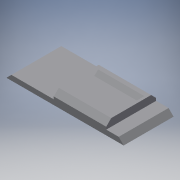
# Autodesk Inventor part: deksel token Nieuw bevestiging uitwendig
Saved by Autodesk Inventor 2018.3 (Build 223284000, 284)
## iProperties
Created: 2020-11-30
Part Number: deksel token Nieuw bevestiging uitwendig
Material: Generic
Document SubType Name: Modeling
Designer: Olivi
Density: 1 g/cm^3
Appearance: Default
Author: Olivi
## iProperties of the stored document deksel token Nieuw bevestiging uitwendig_3DPrint.ipt
Created: 2021-01-08
Part Number: deksel token Nieuw bevestiging uitwendig_3DPrint
Material: Generic
Document SubType Name: Modeling
Designer: daanv
Density: 1 g/cm^3
Appearance: Default
Author: daanv
Autodesk Inventor part; units mm, degrees
ref_plane "YZ Plane" through (0, 0, 0) normal (1, 0, 0) x (0, 1, 0)
ref_plane "XZ Plane" through (0, 0, 0) normal (0, 1, 0) x (-1, 0, 0)
ref_plane "XY Plane" through (0, 0, 0) normal (0, 0, 1) x (1, 0, 0)
sketch "Sketch1" plane through (0, 0, 0) normal (0, 0, 1) x (1, 0, 0)
  line L0 (0, 0) -> (43, 0)
  line L1 (43, 0) -> (43, 20)
  line L2 (43, 20) -> (0, 20)
  line L3 (0, 20) -> (0, 0)
  dimension "d0" = 43
  dimension "d1" = 20
  constraints: 8 end point, 2 parallel, 1 horizontal, 1 perpendicular
  measures "d0" distance of L2.end L1.end
  measures "d1" distance of L1.end L0.end
extrude "Extrusion1" add sketch "Sketch1" along normal blind 2
sketch "Sketch2" plane through (0, 0, 0) normal (0, -1, 0) x (1, 0, 0)
  line L0 (43, 0) -> (43, 2) projected
  line L1 (0, 0) -> (0, 2) projected
  line L2 (0, 0) -> (-2, 0)
  line L3 (-2, 0) -> (0, 2)
  line L4 (43, 0) -> (45, 0)
  line L5 (45, 0) -> (43, 2)
  dimension "d4" = 2
  dimension "d5" = 2
  constraints: 8 end point, 2 horizontal
  measures "d4" distance of L1.start L2.end
  measures "d5" distance of L0.start L4.end
extrude "Extrusion2" add sketch "Sketch2" against normal blind 20
sketch "Sketch6" plane through (0, 0, 2) normal (0, 0, 1) x (1, 0, 0)
  line L0 (0, 0) -> (43, 0) projected
  line L1 (43, 0) -> (43, 20) projected
  line L2 (43, 20) -> (0, 20) projected
  line L3 (17, 3.75) -> (37, 3.75)
  line L4 (37, 3.75) -> (37, 16.25)
  line L5 (37, 16.25) -> (17, 16.25)
  line L6 (17, 16.25) -> (17, 3.75)
  line L7 (17, 3.75) -> (37, 3.75)
  line L8 (37, 3.75) -> (37, 0)
  line L9 (37, 0) -> (17, 0)
  line L10 (17, 0) -> (17, 3.75)
  line L11 (17, 16.25) -> (37, 16.25)
  line L12 (37, 16.25) -> (37, 20)
  line L13 (37, 20) -> (17, 20)
  line L14 (17, 20) -> (17, 16.25)
  dimension "d47" = 20
  dimension "d48" = 12.5
  dimension "d49" = 3.75
  dimension "d50" = 3.75
  dimension "d51" = 6
  dimension "d52" = 6
  constraints: 24 end point, 6 parallel, 3 horizontal, 3 perpendicular, 3 point on line
  measures "d47" distance of L5.end L4.end
  measures "d48" distance of L4.end L3.end
  measures "d49" distance between parallel lines of L0 L3
  measures "d50" distance between parallel lines of L2 L5
  measures "d51" distance between parallel lines of L1 L4
  measures "d52" distance between parallel lines of L1 L12
extrude "Extrusion6" add sketch "Sketch6" along normal blind 3 contours L10 L3 L8 L0 | L14 L2 L12 L5
sketch "Sketch7" plane through (37, 0, 2) normal (1, 0, 0) x (0, 0, -1)
  line L0 (0, 3.75) -> (-3, 3.75) projected
  line L1 (-3, 3.75) -> (-3, 0) projected
  line L2 (-3, 3.75) -> (-1.5009, 2.2509)
  line L3 (-3, 3.75) -> (-0.88, 3.75) construction
  line L4 (-1.5009, 2.2509) -> (0, 3.75)
  point P0 (2, 0)
  dimension "d55" = 2.12
  dimension "d56" = 45
  constraints: 6 end point, 1 equal length, 1 horizontal
  measures "d55" distance of L0.end L2.end
  measures "d56" angle of L2 L3
extrude "Extrusion7" cut sketch "Sketch7" against normal up to next
sketch "Sketch8" plane through (37, 16.25, 2) normal (1, 0, 0) x (0, 0, -1)
  line L0 (0, 0) -> (-3, 0) projected
  line L1 (-3, 0) -> (-1.5009, 1.4991)
  line L2 (-3, 0) -> (-0.88, 0) construction
  line L3 (-1.5009, 1.4991) -> (0, 0)
  point P0 (2, -16.25)
  dimension "d59" = 2.12
  dimension "d60" = 45
  constraints: 6 end point, 1 equal length, 1 horizontal
  measures "d59" distance of L0.end L1.end
  measures "d60" angle of L2 L1
extrude "Extrusion8" cut sketch "Sketch8" against normal up to next
chamfer "Chamfer7" distance 2 angle 45 1 edges at (27, 0, 5)
chamfer "Chamfer8" distance 2 angle 45 1 edges at (27, 20, 5)
sketch "Sketch9" plane through (0, 0, 2) normal (0, 0, 1) x (1, 0, 0)
  line L0 (37, 0) -> (43, 0) projected
  line L1 (37, 20) -> (38, 20)
  line L2 (38, 20) -> (38, 0)
  line L3 (38, 0) -> (37, 0)
  line L4 (37, 0) -> (37, 20)
  dimension "d69" = 1
  constraints: 8 end point, 2 parallel, 1 horizontal, 1 perpendicular, 1 point on line
  measures "d69" distance of L2.end L3.end
extrude "Extrusion9" add sketch "Sketch9" along normal blind 3
chamfer "Chamfer9" distance 2 angle 45 1 edges at (37.5, 0, 5)
chamfer "Chamfer10" distance 2 angle 45 1 edges at (37.5, 20, 5)
body "Solid1"
